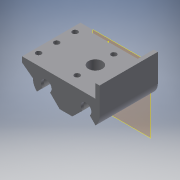
# Autodesk Inventor part: X Carriage
Saved by Autodesk Inventor 2016 (Build 200138000, 138)
## iProperties
Created: 2016-05-27
Part Number: X Carriage
Material: Generic
Document SubType Name: Modeling
Designer: Scott
Density: 1 g/cm^3
Appearance: Default
Author: Scott
Autodesk Inventor part; units mm, degrees
ref_plane "YZ Plane" through (0, 0, 0) normal (1, 0, 0) x (0, 1, 0)
ref_plane "XZ Plane" through (0, 0, 0) normal (0, 1, 0) x (-1, 0, 0)
ref_plane "XY Plane" through (0, 0, 0) normal (0, 0, 1) x (1, 0, 0)
ref_plane "Work Plane1" through (0, 0, 0) normal (0, 0, 1) x (1, 0, 0)
sketch "Sketch1" plane through (0, 0, 0) normal (0, 0, 1) x (1, 0, 0)
  circle A0 centre (31.455, -10.16) radius 4 projected
  circle A1 centre (-6.055, -10.16) radius 4 projected
  circle A2 centre (-6.055, -10.16) radius 8
  circle A3 centre (31.455, -10.16) radius 8
  circle A4 centre (-6.055, -10.16) radius 12.7
  circle A5 centre (31.455, -10.16) radius 12.7
  line L0 (-6.055, 2.54) -> (31.455, 2.54)
  line L1 (-6.055, -22.86) -> (31.455, -22.86)
  point P0 (0, 0)
  dimension "d0" = 16
  dimension "d1" = 16
  dimension "d2" = 25.4
  dimension "d3" = 25.4
  constraints: 4 centre point, 4 coincident, 4 end point, 4 point on circle, 2 tangent
  measures "d0" diameter of A2
  measures "d1" diameter of A3
  measures "d2" diameter of A4
  measures "d3" diameter of A5
extrude "Extrusion1" add sketch "Sketch1" along normal blind 24 contours A4 | A4 L0 A5 L1 | A5
sketch "Sketch2" plane through (-6.055, 2.54, 0) normal (0, 1, 0) x (1, 0, 0)
  point P0 (6.055, 0)
sketch "Sketch3" plane through (0, 0, 24) normal (0, 0, 1) x (1, 0, 0)
  circle A0 centre (31.455, -10.16) radius 8 projected
  circle A1 centre (-6.055, -10.16) radius 8 projected
  line L0 (-6.055, -22.86) -> (31.455, -22.86) projected
  arc A2 (31.455, -22.86) -> (31.455, 2.54) centre (31.455, -10.16) ccw projected
  line L1 (31.455, 2.54) -> (-6.055, 2.54) projected
  arc A3 (-6.055, 2.54) -> (-6.055, -22.86) centre (-6.055, -10.16) ccw projected
  circle A4 centre (-6.055, -10.16) radius 5
  circle A5 centre (31.455, -10.16) radius 5
  point P0 (0, 0)
  dimension "d6" = 10
  dimension "d7" = 10
  constraints: 2 centre point, 2 coincident
  measures "d6" diameter of A4
  measures "d7" diameter of A5
extrude "Extrusion2" add sketch "Sketch3" along normal blind 2 contours A0 | A1 | A3 L1 A2 L0
sketch "Sketch4" plane through (0, 0, 26) normal (0, 0, 1) x (1, 0, 0)
  circle A0 centre (-6.055, -10.16) radius 5 projected
  circle A1 centre (31.455, -10.16) radius 5 projected
  line L0 (-6.055, -22.86) -> (31.455, -22.86) projected
  arc A2 (31.455, -22.86) -> (31.455, 2.54) centre (31.455, -10.16) ccw projected
  line L1 (31.455, 2.54) -> (-6.055, 2.54) projected
  arc A3 (-6.055, 2.54) -> (-6.055, -22.86) centre (-6.055, -10.16) ccw projected
  circle A4 centre (-6.055, -10.16) radius 8 projected
  circle A5 centre (31.455, -10.16) radius 8 projected
  point P0 (0, 0)
extrude "Extrusion3" add sketch "Sketch4" along normal blind 24 contours A3 L1 A2 L0
sketch "Sketch5" plane through (-6.055, 2.54, 0) normal (0, 1, 0) x (1, 0, 0)
  line L0 (37.51, 0) -> (0, 0) projected
  line L1 (0, 0) -> (0, -50) projected
  line L2 (37.51, -50) -> (0, -50) projected
  line L3 (37.51, 0) -> (37.51, -50) projected
  circle A0 centre (18.755, -25) radius 6.5
  point P0 (6.055, 0)
  dimension "d12" = 13
  constraints: 1 centre point
  measures "d12" diameter of A0
extrude "Extrusion4" cut sketch "Sketch5" against normal blind 36.7 contours A0
sketch "Sketch6" plane through (0, 0, 50) normal (0, 0, 1) x (1, 0, 0)
  circle A0 centre (31.455, -10.16) radius 8 projected
  circle A1 centre (-6.055, -10.16) radius 8 projected
  line L0 (-6.055, -22.86) -> (31.455, -22.86) projected
  arc A2 (31.455, -22.86) -> (31.455, 2.54) centre (31.455, -10.16) ccw projected
  line L1 (31.455, 2.54) -> (-6.055, 2.54) projected
  arc A3 (-6.055, 2.54) -> (-6.055, -22.86) centre (-6.055, -10.16) ccw projected
  circle A4 centre (-6.055, -10.16) radius 8 projected
  line L2 (-11.7741, -15.7539) -> (-14.9136, -19.2603)
  arc A5 (-6.055, 2.54) -> (-6.055, -22.86) centre (-6.055, -10.16) ccw projected
  line L3 (-11.7741, -15.7539) -> (-7.0676, -15.7539) construction
  line L4 (-0.4611, -15.8791) -> (6.5197, -22.86)
  line L5 (-6.055, -22.86) -> (31.455, -22.86) projected
  line L6 (-0.4611, -15.8791) -> (9.4113, -15.8791) construction
  circle A6 centre (31.455, -10.16) radius 8 projected
  line L7 (25.7359, -15.7539) -> (18.4706, -22.86)
  line L8 (37.0489, -15.8791) -> (40.3353, -19.2391)
  arc A7 (31.455, -22.86) -> (31.455, 2.54) centre (31.455, -10.16) ccw projected
  line L9 (25.7359, -15.7539) -> (31.455, -10.16)
  line L10 (31.455, -10.16) -> (37.0489, -15.8791)
  line L11 (-0.4611, -15.8791) -> (-6.055, -10.16)
  line L12 (-6.055, -10.16) -> (-11.7741, -15.7539)
  point P0 (0, 0)
  dimension "d16" = 45
  constraints: 20 end point, 11 point on circle, 4 perpendicular, 2 equal length, 2 horizontal, 2 point on line, 1 parallel
  measures "d16" angle of L4 L6
extrude "Extrusion5" cut sketch "Sketch6" against normal blind 96.8375 contours L9 L10 A0 | A0 L8 A2 L0 L7 | L0 A3 L2 A1 L4 | A1 L12 L11 picked at (30.2186, -15.3136) picked at (-7.2914, -15.3136)
sketch "Sketch7" plane through (0, 0, 0) normal (0, 0, -1) x (-1, 0, 0)
  line L0 (11.7741, -15.7539) -> (14.9136, -19.2603) projected
  arc A0 (14.9136, -19.2603) -> (6.055, 2.54) centre (6.055, -10.16) ccw projected
  line L1 (-31.455, 2.54) -> (6.055, 2.54) projected
  arc A1 (-31.455, 2.54) -> (-40.3353, -19.2391) centre (-31.455, -10.16) ccw projected
  line L2 (-40.3353, -19.2391) -> (-37.0489, -15.8791) projected
  arc A2 (-25.7359, -15.7539) -> (-37.0489, -15.8791) centre (-31.455, -10.16) ccw projected
  line L3 (-25.7359, -15.7539) -> (-18.4706, -22.86) projected
  line L4 (-6.5197, -22.86) -> (-18.4706, -22.86) projected
  line L5 (-6.5197, -22.86) -> (0.4611, -15.8791) projected
  arc A3 (11.7741, -15.7539) -> (0.4611, -15.8791) centre (6.055, -10.16) ccw projected
  arc A4 (-25.7359, -15.7539) -> (-37.0489, -15.8791) centre (-31.455, -10.16) ccw projected
  arc A5 (-27.8805, -13.6562) -> (-34.9512, -13.7345) centre (-31.455, -10.16) ccw projected
  line L6 (-37.0489, -15.8791) -> (-34.9512, -13.7345) projected
  arc A6 (-27.8805, -13.6562) -> (-34.9512, -13.7345) centre (-31.455, -10.16) ccw projected
  line L7 (-27.8805, -13.6562) -> (-25.7359, -15.7539) projected
  arc A7 (-25.7359, -15.7539) -> (-37.0489, -15.8791) centre (-31.455, -10.16) ccw projected
  line L8 (9.6295, -13.6562) -> (11.7741, -15.7539) projected
  arc A8 (11.7741, -15.7539) -> (0.4611, -15.8791) centre (6.055, -10.16) ccw projected
  line L9 (0.4611, -15.8791) -> (2.5588, -13.7345) projected
  arc A9 (9.6295, -13.6562) -> (2.5588, -13.7345) centre (6.055, -10.16) ccw projected
  point P0 (0, 0)
extrude "Extrusion6" add sketch "Sketch7" along normal blind 2.54
sketch "Sketch8" plane through (0, 0, 50) normal (0, 0, 1) x (1, 0, 0)
  line L0 (-14.9136, -19.2603) -> (-11.7741, -15.7539) projected
  arc A0 (-0.4611, -15.8791) -> (-11.7741, -15.7539) centre (-6.055, -10.16) ccw projected
  line L1 (-0.4611, -15.8791) -> (6.5197, -22.86) projected
  line L2 (6.5197, -22.86) -> (18.4706, -22.86) projected
  line L3 (18.4706, -22.86) -> (25.7359, -15.7539) projected
  arc A1 (37.0489, -15.8791) -> (25.7359, -15.7539) centre (31.455, -10.16) ccw projected
  line L4 (37.0489, -15.8791) -> (40.3353, -19.2391) projected
  arc A2 (40.3353, -19.2391) -> (31.455, 2.54) centre (31.455, -10.16) ccw projected
  line L5 (31.455, 2.54) -> (-6.055, 2.54) projected
  arc A3 (-6.055, 2.54) -> (-14.9136, -19.2603) centre (-6.055, -10.16) ccw projected
  line L6 (-11.7741, -15.7539) -> (-9.6295, -13.6562) projected
  arc A4 (-2.5588, -13.7345) -> (-9.6295, -13.6562) centre (-6.055, -10.16) ccw projected
  line L7 (-2.5588, -13.7345) -> (-0.4611, -15.8791) projected
  arc A5 (-0.4611, -15.8791) -> (-11.7741, -15.7539) centre (-6.055, -10.16) ccw projected
  line L8 (34.9512, -13.7345) -> (37.0489, -15.8791) projected
  arc A6 (37.0489, -15.8791) -> (25.7359, -15.7539) centre (31.455, -10.16) ccw projected
  line L9 (25.7359, -15.7539) -> (27.8805, -13.6562) projected
  arc A7 (34.9512, -13.7345) -> (27.8805, -13.6562) centre (31.455, -10.16) ccw projected
  point P0 (0, 0)
extrude "Extrusion7" add sketch "Sketch8" along normal blind 2.54
sketch "Sketch9" plane through (-6.055, 2.54, -2.54) normal (0, 1, 0) x (1, 0, 0)
  line L0 (50.21, 0) -> (50.21, -55.08) projected
  line L1 (37.51, 0) -> (37.51, -55.08) projected
  line L2 (50.21, 0) -> (37.51, 0) projected
  line L3 (37.51, -55.08) -> (50.21, -55.08) projected
  point P0 (6.055, -2.54)
  point P1 (46.3903, 0)
  point P2 (46.3903, -55.08)
extrude "Extrusion8" add sketch "Sketch9" against normal up to next
sketch "Sketch10" plane through (-6.055, 2.54, 52.54) normal (0, 1, 0) x (1, 0, 0)
  line L0 (5, 0) -> (-5, 0) projected
  line L1 (-8, 52.54) -> (8, 52.54) projected
  line L2 (-5.7191, 52.54) -> (-5.7191, 2.54)
  line L3 (-5.7191, 52.54) -> (44.2809, 52.54) construction
  circle A0 centre (18.755, 27.54) radius 6.5 projected
  line L4 (0, 55.08) -> (0, 0) projected
  line L5 (50.21, 0) -> (0, 0) projected
  line L6 (50.21, 55.08) -> (50.21, 0) projected
  line L7 (0, 55.08) -> (50.21, 55.08) projected
  line L8 (-8.8586, 55.08) -> (-8.8586, 0) projected
  line L9 (0, 0) -> (-8.8586, 0) projected
  line L10 (0, 55.08) -> (0, 0) projected
  line L11 (-8.8586, 55.08) -> (0, 55.08) projected
  point P0 (6.055, 52.54)
  point P1 (-3.5745, 0)
  point P2 (3.4962, 0)
  point P3 (5.5939, 52.54)
  dimension "d25" = 90
  constraints: 4 end point, 1 horizontal, 1 perpendicular
  measures "d25" angle of L2 L3
extrude "Extrusion9" add sketch "Sketch10" against normal up to next contours L0 L9 L8 L11 L4
sketch "Sketch11" plane through (44.155, 2.54, 52.54) normal (0, 1, 0) x (1, 0, 0)
  line L0 (0, 55.08) -> (0, 0) projected
  line L1 (-4.7, 52.54) -> (-4.7, 28.54) projected
  line L2 (0, 55.08) -> (0, 0) projected
  line L3 (0, 0) -> (-59.0686, 0) projected
  line L4 (0, 55.08) -> (-3.81, 55.08)
  line L5 (-3.81, 55.08) -> (-3.81, 0)
  line L6 (-3.81, 0) -> (0, 0)
  line L7 (0, 0) -> (0, 55.08)
  point P0 (-44.155, 52.54)
  dimension "d28" = 3.81
  constraints: 8 end point, 2 parallel, 1 horizontal, 1 perpendicular, 1 point on line
  measures "d28" distance of L6.end L5.end
extrude "Extrusion10" add sketch "Sketch11" along normal blind 12.7
sketch "Sketch12" plane through (-14.9136, 2.54, 52.54) normal (0, 1, 0) x (1, 0, 0)
  line L0 (55.2586, 0) -> (55.2586, 55.08) projected
  line L1 (55.2586, 55.08) -> (0, 55.08) projected
  line L2 (0, 55.08) -> (0, 0) projected
  line L3 (55.2586, 0) -> (0, 0) projected
  circle A0 centre (27.6136, 27.54) radius 6.5 projected
  circle A1 centre (27.6136, 27.54) radius 6.5 projected
  line L4 (27.4755, 34.0385) -> (27.4755, 55.08)
  line L5 (33.3842, 55.08) -> (21.4334, 55.08) projected
  line L6 (27.4755, 34.0385) -> (48.517, 34.0385) construction
  line L7 (27.4782, 21.0414) -> (27.4782, 0)
  line L8 (55.2586, 0) -> (0, 0) projected
  line L9 (27.4782, 21.0414) -> (48.5196, 21.0414) construction
  circle A2 centre (27.6293, 44.9428) radius 2.54
  circle A3 centre (27.4782, 10.5207) radius 2.54
  point P0 (14.9136, 52.54)
  dimension "d31" = 90
  dimension "d32" = 90
  dimension "d33" = 5.08
  dimension "d34" = 5.08
  constraints: 8 end point, 4 point on circle, 2 centre point, 2 horizontal, 2 perpendicular, 2 point on line, 1 midpoint
  measures "d31" angle of L6 L4
  measures "d32" angle of L7 L9
  measures "d33" diameter of A2
  measures "d34" diameter of A3
extrude "Extrusion11" cut sketch "Sketch12" against normal blind 76.2 contours A3 L7 | L7 A3 | A2 L4 | L4 A2
sketch "Sketch13" plane through (-14.9136, 2.54, 52.54) normal (0, 1, 0) x (1, 0, 0)
  line L0 (0, 0) -> (0, 55.08) projected
  line L1 (0, 55.08) -> (0, 55.08) projected
  line L2 (0, 55.08) -> (0, 0) projected
  line L3 (0, 0) -> (0, 0) projected
  line L4 (-3.8414, 55.08) -> (-3.8414, 0) projected
  line L5 (0, 55.08) -> (-3.8414, 55.08)
  line L6 (-3.8414, 55.08) -> (-3.8414, 0)
  line L7 (-3.8414, 0) -> (0, 0)
  line L8 (0, 0) -> (0, 55.08)
  point P0 (14.9136, 52.54)
  constraints: 8 end point, 2 parallel, 1 horizontal, 1 perpendicular
extrude "Extrusion12" add sketch "Sketch13" against normal up to surface round surface about axis through (-6.055, -10.16, 0) along (0, 0, 1) radius 12.7 far side no
sketch "Sketch14" plane through (40.345, 2.54, 52.54) normal (0, 1, 0) x (1, 0, 0)
  circle A0 centre (-27.7805, 10.5207) radius 2.54 projected
  circle A1 centre (-27.6293, 44.9428) radius 2.54 projected
  line L0 (0, 0) -> (0, 55.08) projected
  line L1 (0, 55.08) -> (-59.1, 55.08) projected
  line L2 (-59.1, 55.08) -> (-59.1, 0) projected
  line L3 (0, 0) -> (-59.1, 0) projected
  circle A2 centre (-27.645, 27.54) radius 6.5 projected
  line L4 (-59.1, 55.08) -> (-69.26, 55.08)
  line L5 (-69.26, 55.08) -> (-69.26, 0)
  line L6 (-69.26, 0) -> (-59.1, 0)
  line L7 (-59.1, 0) -> (-59.1, 55.08)
  point P0 (-40.345, 52.54)
  dimension "d39" = 10.16
  constraints: 8 end point, 2 parallel, 1 horizontal, 1 perpendicular
  measures "d39" distance of L6.end L5.end
extrude "Extrusion13" add sketch "Sketch14" against normal blind 5.08 contours L6 L5 L4 L2
sketch "Sketch15" plane through (0, 0, -2.54) normal (0, 0, -1) x (-1, 0, 0)
  line L0 (-40.345, 2.54) -> (28.915, 2.54) projected
  line L1 (-40.345, 2.54) -> (-40.345, 15.24) projected
  line L2 (-44.155, 15.24) -> (-40.345, 15.24) projected
  line L3 (-44.155, -10.16) -> (-44.155, 15.24) projected
  arc A0 (-44.155, -10.16) -> (-40.3353, -19.2391) centre (-31.455, -10.16) ccw projected
  line L4 (-40.3353, -19.2391) -> (-34.9512, -13.7345) projected
  arc A1 (-27.8805, -13.6562) -> (-34.9512, -13.7345) centre (-31.455, -10.16) ccw projected
  line L5 (-27.8805, -13.6562) -> (-18.4706, -22.86) projected
  line L6 (-18.4706, -22.86) -> (-6.5197, -22.86) projected
  line L7 (-6.5197, -22.86) -> (0.4611, -15.8791) projected
  line L8 (0.4611, -15.8791) -> (2.5588, -13.7345) projected
  arc A2 (9.6295, -13.6562) -> (2.5588, -13.7345) centre (6.055, -10.16) ccw projected
  line L9 (9.6295, -13.6562) -> (11.7741, -15.7539) projected
  line L10 (11.7741, -15.7539) -> (14.9136, -19.2603) projected
  arc A3 (14.9136, -19.2603) -> (18.755, -10.16) centre (6.055, -10.16) ccw projected
  line L11 (18.755, -2.54) -> (18.755, -10.16) projected
  line L12 (28.915, -2.54) -> (18.755, -2.54) projected
  line L13 (28.915, 2.54) -> (28.915, -2.54) projected
  line L14 (18.755, -2.54) -> (18.755, -10.16) projected
  line L15 (28.915, -2.54) -> (18.755, -2.54) projected
  line L16 (18.755, -10.16) -> (28.915, -2.54)
  point P0 (0, 0)
  constraints: 2 end point
extrude "Extrusion14" add sketch "Sketch15" against normal blind 2.54 contours L16 L11 L12
sketch "Sketch16" plane through (0, 0, 52.54) normal (0, 0, 1) x (1, 0, 0)
  line L0 (-18.755, -2.54) -> (-18.755, -10.16) projected
  line L1 (-18.755, -2.54) -> (-28.915, -2.54) projected
  line L2 (-18.755, -10.16) -> (-28.915, -2.54)
  point P0 (0, 0)
  constraints: 2 end point
extrude "Extrusion15" add sketch "Sketch16" against normal blind 2.54
sketch "Sketch17" plane through (40.345, 2.54, 52.54) normal (0, 1, 0) x (1, 0, 0)
  circle A0 centre (-27.7805, 10.5207) radius 2.54 projected
  circle A1 centre (-27.6293, 44.9428) radius 2.54 projected
  line L0 (0, 0) -> (0, 55.08) projected
  line L1 (0, 55.08) -> (-69.26, 55.08) projected
  line L2 (-69.26, 55.08) -> (-69.26, 0) projected
  line L3 (0, 0) -> (-69.26, 0) projected
  circle A2 centre (-27.645, 27.54) radius 6.5 projected
  line L4 (-59.1, 2.54) -> (-59.1, 52.54) projected
  line L5 (-59.1, 55.08) -> (-59.1, 52.54) projected
  line L6 (-69.26, 52.54) -> (-59.1, 52.54) projected
  line L7 (-59.1, 52.54) -> (-69.26, 52.54)
  circle A3 centre (-64.18, 44.9428) radius 2.54
  circle A4 centre (-64.18, 10.5207) radius 2.54
  line L8 (-27.645, 27.54) -> (-64.18, 27.54)
  circle A5 centre (-64.18, 27.54) radius 2.54
  point P0 (-40.345, 52.54)
  dimension "d46" = 5.08
  dimension "d47" = 5.08
  dimension "d48" = 5.08
  constraints: 4 end point, 3 centre point, 1 coincident, 1 collinear, 1 horizontal
  measures "d46" diameter of A3
  measures "d47" diameter of A4
  measures "d48" diameter of A5
extrude "Extrusion16" cut sketch "Sketch17" against normal blind 13.6525 contours A3 | A4 | A5
body "Solid1"
